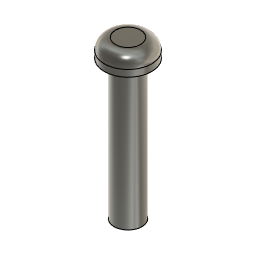
螺钉M5_25 v1 (Autodesk Fusion 360 design; units mm, degrees)
Autodesk Fusion 360 part; units mm, degrees
sketch "草图1" plane through (0, 0, 0) normal (0, 0, 1) x (1, 0, 0)
  circle A0 centre (0, 0) radius 4.25
  dimension "d1" = 8.5
  constraint coincident A0.centre origin
  measures "d1" diameter of A0
extrude "拉伸1" add sketch "草图1" along normal blind 3.2
fillet "圆角1" radius 2 1 edges at (-3.9624, -1.5369, 3.2)
sketch "草图2" plane through (0, 0, 0) normal (0, 0, -1) x (1, 0, 0)
  circle A0 centre (0, 0) radius 4.25
  circle A1 centre (0, 0) radius 2.5
  dimension "d6" = 5
  constraint coincident A0.centre A1.centre
  measures "d6" diameter of A1
extrude "拉伸2" add sketch "草图2" along normal blind 25 contours A1
